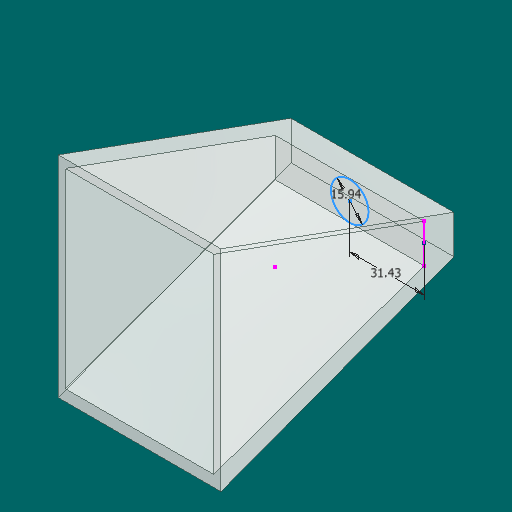
# Autodesk Inventor part: CamBody
Saved by Autodesk Inventor 2025.2 (Build 292293000, 293)
## iProperties
Created: 2025-04-19
Part Number: CamBody
Material: Generic
Document SubType Name: Modeling
Designer: Matt Caldwell
Density: 1 g/cm^3
Appearance: Default
Author: Matt Caldwell
Autodesk Inventor part; units mm, degrees
ref_plane "YZ Plane" through (0, 0, 0) normal (1, 0, 0) x (0, 1, 0)
ref_plane "XZ Plane" through (0, 0, 0) normal (0, 1, 0) x (-1, 0, 0)
ref_plane "XY Plane" through (0, 0, 0) normal (0, 0, 1) x (1, 0, 0)
ref_plane "Work Plane1" through (0, 32.027, -88.9) normal (0, 0, -1) x (-1, 0, 0)
sketch "Sketch5" plane through (0, 32.027, -88.9) normal (0, 0, -1) x (-1, 0, 0)
  circle A0 centre (-31.43, 7.9375) radius 7.97
  line L0 (-62.86, 0) -> (-62.86, 16.266) projected
  point P0 (0, -32.027)
  point P1 (-62.86, 8.133)
  dimension "d28" = 15.94
  dimension "d29" = 31.43
  constraints: 1 centre point, 1 midpoint
  measures "d28" diameter of A0
  measures "d29" horizontal distance of point (-62.86, 8.133) A0.centre
ref_plane "Work Plane2" through (62.86, 0, 0) normal (1, 0, 0) x (0, 0, -1)
sketch "Sketch7" plane through (62.86, 0, 0) normal (1, 0, 0) x (0, 0, -1)
  line L0 (0, 80.65) -> (0, 0) projected
  line L1 (0, 0) -> (88.9, 32.027) projected
  line L2 (0, 0) -> (88.9, 32.027)
  line L3 (88.9, 32.027) -> (88.9, 48.293) projected
  line L4 (88.9, 32.027) -> (88.9, 48.293)
  line L5 (88.9, 48.293) -> (0, 80.65) projected
  line L6 (88.9, 48.293) -> (0, 80.65)
  line L7 (0, 80.65) -> (0, 84.1375)
  line L8 (0, 84.1375) -> (98.4818, 48.293)
  line L9 (98.4818, 48.293) -> (98.4818, 32.027)
  line L10 (98.4818, 32.027) -> (0, -4.7625)
  line L11 (0, -4.7625) -> (0, 0)
  constraints: 16 end point, 4 parallel, 3 collinear, 1 point on line
extrude "Shell" add sketch "Sketch7" against normal blind 62.86 contours L7 L8 L9 L10 L11 L1 L3 L5
sketch "Sketch8" plane through (62.86, 0, 0) normal (1, 0, 0) x (0, 0, -1)
  line L0 (98.4818, 48.293) -> (0, 84.1375) projected
  line L1 (0, -4.7625) -> (98.4818, 32.027) projected
  line L2 (0, 84.1375) -> (0, -4.7625)
  line L3 (98.4818, 32.027) -> (98.4818, 48.293) projected
  line L4 (0, -4.7625) -> (98.4818, 32.027)
  line L5 (98.4818, 32.027) -> (98.4818, 48.293)
  line L6 (98.4818, 48.293) -> (0, 84.1375)
  point P0 (0, 0)
  constraints: 8 end point, 1 collinear, 1 vertical
extrude "Extrusion4" add sketch "Sketch8" along normal blind 3
sketch "Sketch9" plane through (0, 0, 0) normal (-1, 0, 0) x (0, 0, 1)
  line L0 (0, 80.65) -> (0, 84.1375) projected
  line L1 (0, 84.1375) -> (-98.4818, 48.293) projected
  line L2 (0, 84.1375) -> (-98.4818, 48.293)
  line L3 (-98.4818, 48.293) -> (-98.4818, 32.027) projected
  line L4 (-98.4818, 48.293) -> (-98.4818, 32.027)
  line L5 (-98.4818, 32.027) -> (0, -4.7625)
  line L6 (0, -4.7625) -> (0, 84.1375)
  point P0 (0, 0)
  constraints: 8 end point, 2 collinear, 1 parallel
extrude "Extrusion5" add sketch "Sketch9" along normal blind 3
body "Solid2"
